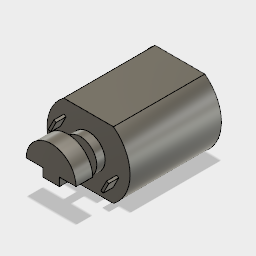
Vibe Motor v4 (Autodesk Fusion 360 design; units mm, degrees)
Autodesk Fusion 360 part; units mm, degrees
sketch "Sketch1" plane through (0, 0, 0) normal (0, 0, 1) x (1, 0, 0)
  circle A0 centre (0, 0) radius 5
  line L0 (-8, 4) -> (9, 4)
  line L1 (-8, -4) -> (9, -4)
  line L2 (-8, -4) -> (-8, 4)
  line L3 (-8, 0) -> (8, 0)
  dimension "d1" = 10
  dimension "d2" = 8
  constraint coincident A0.centre origin
  constraint horizontal L0
  constraint horizontal L1
  constraint perpendicular L0 L2
  constraint midpoint L2 A0.centre
  constraint perpendicular L2 L3
  constraint midpoint L3 A0.centre
  measures "d1" diameter of A0
extrude "Extrude1" add sketch "Sketch1" along normal blind 11 contours A0 L0 L3 | A0 L1 L3
sketch "Sketch2" plane through (0, 0, 0) normal (0, 0, -1) x (-1, 0, 0)
  arc A0 (3, -4) -> (3, 4) centre (0, 0) ccw
  line L0 (3, 4) -> (-3, 4)
  arc A1 (-3, 4) -> (-3, -4) centre (0, 0) ccw
  line L1 (-3, -4) -> (3, -4)
  circle A2 centre (0, 0) radius 2
  circle A3 centre (0, 0) radius 0.5
  dimension "d5" = 4
  dimension "d6" = 1
  constraint concentric A0 A2
  constraint concentric A2 A3
  measures "d5" diameter of A2
  measures "d6" diameter of A3
extrude "Extrude2" add sketch "Sketch2" along normal blind 0.5 contours A2
extrude "Extrude3" add 1 faces at (0.3432, -0.1249, 0) along direction (0, 0, -1) blind 3
sketch "Sketch3" plane through (0, 0, 11) normal (0, 0, 1) x (1, 0, 0)
  arc A0 (-3, 4) -> (-3, -4) centre (0, 0) ccw
  line L0 (-3, -4) -> (3, -4)
  arc A1 (3, -4) -> (3, 4) centre (0, 0) ccw
  line L1 (3, 4) -> (-3, 4)
  circle A2 centre (0, 0) radius 2
  circle A3 centre (0, 0) radius 0.5
  circle A4 centre (0, 0) radius 3.775
  line L2 (3.6401, -4) -> (3.6401, -1)
  line L3 (-3.6401, 4) -> (-3.6401, 1)
  line L4 (-3.6401, 1) -> (-2.9633, 2.3386)
  line L5 (3.6401, -1) -> (2.9633, -2.3386)
  line L6 (-2.9633, 2.3386) -> (-2.6956, 2.2033)
  line L7 (-2.6956, 2.2033) -> (-3.3724, 0.8646)
  line L8 (-3.3724, 0.8646) -> (-3.6401, 1)
  line L9 (3.6401, -1) -> (3.3724, -0.8646)
  line L10 (2.9633, -2.3386) -> (2.6956, -2.2033)
  line L11 (2.6956, -2.2033) -> (3.3724, -0.8646)
  dimension "d11" = 4
  dimension "d12" = 1
  dimension "d13" = 7.55
  dimension "d14" = 3
  dimension "d15" = 3
  dimension "d16" = 1.5
  dimension "d17" = 1.5
  dimension "d18" = 0.3
  dimension "d19" = 0.3
  constraint concentric A0 A2
  constraint concentric A2 A3
  constraint concentric A3 A4
  constraint coincident L0 A0.centre
  constraint coincident A4 A0.centre
  constraint perpendicular L0 L2
  constraint coincident L1 A0.centre
  constraint perpendicular L1 L3
  constraint coincident A4
  constraint perpendicular L4 L6
  constraint perpendicular L6 L7
  constraint perpendicular L7 L8
  constraint perpendicular L5 L9
  constraint perpendicular L5 L10
  constraint perpendicular L9 L11
  measures "d11" diameter of A2
  measures "d12" diameter of A3
  measures "d13" diameter of A4
  measures "d16" distance of A0.centre
  measures "d17" distance of A0.centre
  measures "d18" distance of A0.centre
  measures "d19" distance of A0.centre
extrude "Extrude4" add sketch "Sketch3" along normal blind 1.2 contours L4 L6 L7 L8
extrude "Extrude5" add sketch "Sketch3" along normal blind 1.2 contours L5 L9 L10 L11
extrude "Extrude6" add sketch "Sketch3" along normal blind 1 contours A2
extrude "Extrude7" add sketch "Sketch3" along normal blind 4.5 contours A3
sketch "Sketch4" plane through (0, 0, 15.5) normal (0, 0, 1) x (1, 0, 0)
  circle A0 centre (0, 0) radius 0.5
  circle A1 centre (0, 0) radius 3
  line L0 (1, -1) -> (-1, -1)
  line L1 (-1, -1) -> (-1, 1)
  line L2 (-1, 1) -> (1, 1)
  line L3 (1, 1) -> (1, -1)
  line L4 (1, -1) -> (-1, 1) construction
  line L5 (-1, -1) -> (1, 1) construction
  line L6 (-3, 0) -> (3, 0)
  dimension "d28" = 6
  dimension "d29" = 2
  dimension "d30" = 2
  constraint coincident A0.centre A1.centre
  constraint perpendicular L0 L1
  constraint parallel L0 L2
  constraint parallel L1 L3
  constraint horizontal L0
  constraint coincident L4 A0.centre
  constraint coincident L5 A0.centre
  constraint coincident A1 A0.centre
  constraint perpendicular L1 L6
  measures "d28" diameter of A1
extrude "Extrude8" add sketch "Sketch4" against normal blind 2 contours A0 L0 L1 L3 L6 | A0 L1 L2 L3 L6 | A1 L1 L2 L3 L6
